mine (Autodesk Fusion 360 design; units mm, degrees)
Autodesk Fusion 360 part; units mm, degrees
sketch "Sketch1" plane through (0, 0, 0) normal (1, 0, 0) x (0, 1, 0)
  line L0 (0, 0) -> (-72.8969, -68.4547)
  line L1 (0, 0) -> (100, 0) construction
  line L2 (0, 75) -> (0, -60) construction
  line L3 (0, 0) -> (72.8969, -68.4547)
  line L4 (0, 0) -> (0, 50)
  line L5 (0, 50) -> (3.0581, 0)
  line L6 (0, 50) -> (-3.0581, 0)
  line L7 (0, 0) -> (68.4547, 72.8969) construction
  line L8 (0, 50) -> (70.2321, 54.2956)
  line L9 (0, 50) -> (70.3634, 50) construction
  line L10 (49.8142, 53.0468) -> (50, 0)
  line L11 (70.2321, 54.2956) -> (70.2321, 59.2956)
  line L12 (0, 50) -> (0, 55)
  line L13 (0, 55) -> (70.2321, 59.2956)
  line L14 (50, 0) -> (55, 0.0175)
  line L15 (55, 0.0175) -> (54.7957, 58.3514)
  dimension "d6" = 7
  dimension "d7" = 46.8
  dimension "d8" = 3.5
  dimension "d10" = 5
  dimension "d11" = 5
  dimension "d12" = 5
  constraint horizontal L1
  constraint coincident L0.start L1.start
  constraint vertical L2
  constraint symmetric L0.start L2 L1.start
  constraint symmetric L0.end L2 L3.end
  constraint coincident L2 L4.end
  constraint perpendicular L1 L4
  constraint coincident L1 L5.end
  constraint symmetric L5.start L4 L6.start
  constraint symmetric L4 L5.end L6.end
  constraint perpendicular L3 L7
  constraint horizontal L9
  constraint coincident L7 L10.start
  constraint coincident L8 L10.start
  constraint midpoint L1 L10.end
  constraint perpendicular L9 L11
  constraint parallel L2 L12
  constraint perpendicular L10 L14
  constraint coincident L7 L15.end
  constraint coincident L13 L15.end
  measures "d6" angle of L5 L6
  measures "d7" angle of L0 L2
  measures "d8" angle of L8 L9
  measures "d10" distance of L8.end L11.end
  measures "d11" distance of L4.end L12.end
  measures "d12" distance of L10.end L14.end
revolve "Revolve1" add sketch "Sketch1" angle 360 about axis through (0, 0, 75) along (0, 0, -1) contours L8 L12 L13 L15 | L8 L10 L14 L15
